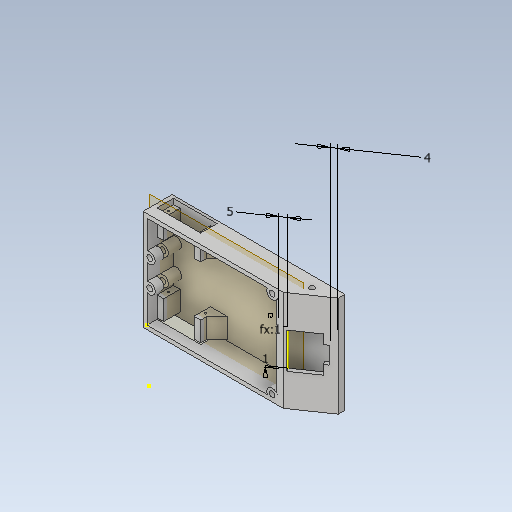
# Autodesk Inventor part: base
Saved by Autodesk Inventor 2020 (Build 240168000, 168)
## iProperties
Created: 2020-01-27
Part Number: base
Material: Ogólne
Document SubType Name: Modeling
Designer: blep
Density: 1 g/cm^3
Appearance: Domyślne
Author: blep
Autodesk Inventor part; units mm, degrees
ref_plane "YZ Plane" through (0, 0, 0) normal (1, 0, 0) x (0, 1, 0)
ref_plane "XZ Plane" through (0, 0, 0) normal (0, 1, 0) x (-1, 0, 0)
sketch "Sketch1" plane through (0, 0, 0) normal (0, 0, 1) x (1, 0, 0)
  line L0 (0, 0) -> (100, 0)
  line L1 (100, 0) -> (100, 70)
  line L2 (100, 70) -> (0, 70)
  line L3 (0, 70) -> (0, 0)
  line L4 (-3, 73) -> (103, 73)
  line L5 (103, 73) -> (103, -3)
  line L6 (103, -3) -> (-3, -3)
  line L7 (-3, -3) -> (-3, 73)
  line L8 (100, 0) -> (103, 0)
  line L9 (100, 70) -> (103, 70)
  dimension "d0" = 100
  dimension "d1" = 70
  dimension "d2" = 3
  constraints: 20 end point, 4 parallel, 3 perpendicular, 2 horizontal, 2 point on line, 3 other
  measures "d0" distance of L2.end L1.end
  measures "d1" distance of L1.end L0.end
  measures "d2" distance between parallel lines of L2 L4
extrude "Extrusion1" add sketch "Sketch1" against normal blind 2
extrude "Extrusion2" add sketch "Sketch1" along normal blind 20 contours L0 L8 L5 L6 L7 L4 L9 L2 L3 | L1 L9 L5 L8
sketch "Sketch2" plane through (0, 70, 0) normal (0, -1, 0) x (1, 0, 0)
  line L0 (0, 0) -> (0, 20) projected
  line L1 (100, 0) -> (0, 0) projected
  line L2 (0, 0) -> (33, 0)
  line L3 (33, 0) -> (33, 12.4)
  line L4 (33, 12.4) -> (0, 12.4)
  line L5 (0, 12.4) -> (0, 0)
  line L6 (100, 0) -> (0, 0) projected
  dimension "d7" = 33
  dimension "d8" = 12.4
  constraints: 8 end point, 2 collinear, 2 parallel, 1 horizontal, 1 perpendicular
  measures "d7" distance of L4.end L3.end
  measures "d8" distance of L3.end L2.end
extrude "Extrusion3" cut sketch "Sketch2" along normal through all both and the other way through all
sketch "Sketch3" plane through (0, 0, 0) normal (0, 0, 1) x (1, 0, 0)
  line L0 (33, 1) -> (28, 1) projected
  line L1 (28, 4) -> (28, 1) projected
  line L2 (0, 1) -> (5, 1) projected
  line L3 (5, 4) -> (5, 1) projected
  line L4 (5, 66) -> (5, 69) projected
  line L5 (0, 69) -> (5, 69) projected
  line L6 (33, 69) -> (28, 69) projected
  line L7 (28, 66) -> (28, 69) projected
  line L8 (33, 54) -> (28, 54)
  line L9 (28, 54) -> (28, 69)
  line L10 (28, 69) -> (33, 69)
  line L11 (33, 69) -> (33, 54)
  line L12 (5, 69) -> (0, 69)
  line L13 (0, 69) -> (0, 54)
  line L14 (0, 54) -> (5, 54)
  line L15 (5, 54) -> (5, 69)
  line L16 (0, 73) -> (0, -3) projected
  line L17 (0, 1) -> (5, 1)
  line L18 (5, 1) -> (5, 16)
  line L19 (5, 16) -> (0, 16)
  line L20 (0, 16) -> (0, 1)
  line L21 (33, 16) -> (28, 16)
  line L22 (28, 16) -> (28, 1)
  line L23 (28, 1) -> (33, 1)
  line L24 (33, 1) -> (33, 16)
  point P0 (0, 0)
  dimension "d11" = 15
  dimension "d12" = 15
  dimension "d13" = 15
  dimension "d14" = 15
  constraints: 32 end point, 8 parallel, 7 collinear, 4 horizontal, 4 perpendicular, 1 coincident, 1 point on line
  measures "d11" distance of L10.end L8.start
  measures "d12" distance of L12.end L13.end
  measures "d13" distance of L17.end L18.end
  measures "d14" distance of L23.end L21.start
ref_plane "Work Plane1" through (0, 66, 12.4) normal (0, 0, 1) x (1, 0, 0)
extrude "Extrusion4" add sketch "Sketch3" along normal up to surface (12.4 mm away)
sketch "Sketch4" plane through (28, 69, 0) normal (0, 1, 0) x (1, 0, 0)
  arc A0 (3.1614, -5.45) -> (3.1614, -6.95) centre (2.5, -6.2) ccw projected
  arc A1 (-26.1614, -6.95) -> (-26.1614, -5.45) centre (-25.5, -6.2) ccw projected
  point P0 (-28, 0)
hole "Hole1" at (30.5, 69, 6.2) at (2.5, 69, 6.2) direction (0, -1, 0) diameter 1.5 end through all
sketch "Sketch5" plane through (-3, 73, -2) normal (0, 1, 0) x (1, 0, 0)
  line L0 (106, -22) -> (0, -22) projected
  line L1 (106, -22) -> (106, 0) projected
  line L2 (0, 0) -> (106, 0) projected
  line L3 (106, -22) -> (106, 0) projected
  line L4 (106, -22) -> (130.7184, -5)
  line L5 (130.7184, -5) -> (130.7184, 0)
  line L6 (130.7184, 0) -> (106, 0)
  line L7 (104.4953, -19.3938) -> (127.7184, -3.4222)
  line L8 (127.7184, -3.4222) -> (127.7184, -3)
  line L9 (127.7184, -3) -> (106, -3)
  line L10 (106, -3) -> (106, 0)
  line L11 (106, -22) -> (100.7059, -22)
  line L12 (100.7059, -22) -> (104.4953, -19.3938)
  point P0 (3, -2)
  dimension "d32" = 30
  dimension "d33" = 5
  dimension "d42" = 3
  constraints: 18 end point, 2 collinear, 2 horizontal, 1 vertical, 2 other
  measures "d32" distance of L0.start L4.end
  measures "d33" distance of L4.end L5.end
  measures "d42" distance between parallel lines of L4 L7
extrude "Extrusion5" cut sketch "Sketch1" along normal through all contours L1 L9 L5 L8
extrude "Extrusion6" add sketch "Sketch5" against normal blind 76 contours L0 L12 L7 L1 | L1 L7 L8 L9 L6 L5 L4
extrude "Extrusion7" add sketch "Sketch5" against normal blind 3 contours L1 L7 L8 L9 L6 L5 L4 | L1 L9 L8 L7
sketch "Sketch6" plane through (-3, -3, -2) normal (0, -1, 0) x (1, 0, 0)
  line L0 (0, 0) -> (130.7184, 0) projected
  line L1 (130.7184, 5) -> (130.7184, 0) projected
  line L2 (106, 22) -> (130.7184, 5) projected
  line L3 (106, 22) -> (106, 0) projected
  point P0 (3, 2)
extrude "Extrusion8" add sketch "Sketch6" against normal blind 3
sketch "Sketch7" plane through (103, 0, 1) normal (-1, 0, 0) x (0, 0, 1)
  line L0 (-1, 0) -> (0, 0) projected
  line L1 (0, 70) -> (0, 0) projected
  line L2 (0, 70) -> (-1, 70) projected
  line L3 (-1, 70) -> (-1, 0) projected
  point P0 (-1, 0)
extrude "Extrusion9" cut sketch "Sketch7" against normal blind 21.75
sketch "Sketch8" plane through (127.7184, -3, 3) normal (0.5667, 0, 0.8239) x (0.8239, 0, -0.5667)
  line L0 (-28, 24.5) -> (-8, 24.5)
  line L1 (-8, 24.5) -> (-8, 51.5)
  line L2 (-8, 51.5) -> (-28, 51.5)
  line L3 (-28, 51.5) -> (-28, 24.5)
  line L4 (0, 76) -> (0, 0) projected
  line L5 (-30, 76) -> (0, 76) projected
  line L6 (-30, 0) -> (-30, 76) projected
  line L7 (0, 0) -> (-30, 0) projected
  line L8 (-28, 51.5) -> (-30, 76) construction
  line L9 (-30, 0) -> (-30, 76) construction
  line L10 (-28, 24.5) -> (-30, 0) construction
  line L11 (-8, 31.5) -> (-5, 31.5)
  line L12 (-5, 31.5) -> (-5, 44.5)
  line L13 (-5, 44.5) -> (-8, 44.5)
  line L14 (-8, 44.5) -> (-8, 31.5)
  line L15 (-8, 24.5) -> (-5, 31.5) construction
  line L16 (-5, 44.5) -> (-8, 51.5) construction
  point P0 (-103.5332, 3)
  dimension "d52" = 27
  dimension "d53" = 20
  dimension "d54" = 3
  dimension "d55" = 13
  dimension "d58" = 2
  constraints: 24 end point, 4 parallel, 2 equal length, 2 horizontal, 2 perpendicular, 1 collinear
  measures "d52" distance of L2.end L0.start
  measures "d53" distance of L1.end L2.end
  measures "d54" distance of L13.end L12.end
  measures "d55" distance of L12.end L11.end
  measures "d58" distance between parallel lines of L9 L3
extrude "Extrusion10" cut sketch "Sketch8" against normal blind 3 contours L3 L2 L1 L0 | L1 L13 L12 L11
sketch "Sketch9" plane through (97.7059, 0, 20) normal (-0.5667, 0, -0.8239) x (-0.8239, 0, 0.5667)
  line L0 (-1.3621, 49.5) -> (-33.3621, 49.5)
  line L1 (-33.3621, 49.5) -> (-33.3621, 20.5)
  line L2 (-33.3621, 20.5) -> (-1.3621, 20.5)
  line L3 (-1.3621, 20.5) -> (-1.3621, 49.5)
  line L4 (-6.3621, 48.5) -> (-6.3621, 21.5) projected
  line L5 (-29.3621, 28.5) -> (-29.3621, 41.5) projected
  point P0 (69.1711, 0)
  dimension "d59" = 5
  dimension "d60" = 4
  dimension "d61" = 1
  dimension "d62" = 1
  constraints: 8 end point, 2 parallel, 1 horizontal, 1 perpendicular
  measures "d59" distance between parallel lines of L3 L4
  measures "d60" distance between parallel lines of L5 L1
  measures "d61" distance from line of L4.end L2
  measures "d62" distance from line of L4.start L0
sketch "Sketch10" plane through (0, 0, 20) normal (0, 0, 1) x (1, 0, 0)
  point P0 (0, 0)
sketch "Sketch12" plane through (-3, -3, -2) normal (0, -1, 0) x (1, 0, 0)
  circle A0 centre (14, 8.2) radius 1.0065 construction
  line L0 (14, 8.2) -> (114, 8.2)
  circle A1 centre (114, 8.2) radius 2
  point P0 (3, 2)
  dimension "d67" = 100
  dimension "d68" = 4
  constraints: 2 end point, 1 centre point, 1 coincident, 1 horizontal
  measures "d67" distance of L0.start L0.end
  measures "d68" diameter of A1
extrude "Extrusion12" cut sketch "Sketch12" against normal through all
sketch "Sketch13" plane through (0, 0, 0) normal (0, 0, 1) x (1, 0, 0)
  circle A0 centre (2, 25) radius 2.125
  circle A1 centre (2, 45) radius 2.125
  line L0 (97.7059, 0) -> (0, 0) projected
  line L1 (0, 70) -> (97.7059, 70) projected
  line L2 (0, 0) -> (0, 70) projected
  circle A2 centre (2, 25) radius 4.125
  circle A3 centre (2, 45) radius 4.125
  dimension "d71" = 25
  dimension "d72" = 25
  dimension "d73" = 2
  dimension "d74" = 4.25
  dimension "d75" = 4.25
  dimension "d76" = 2
  dimension "d77" = 2
  dimension "d78" = 2
  constraints: 4 centre point
  measures "d71" distance from line of L0 A0.centre
  measures "d72" distance from line of L1 A1.centre
  measures "d73" distance from line of A0.centre L2
  measures "d74" diameter of A0
  measures "d75" diameter of A1
  measures "d76" distance from line of A1.centre L2
  measures "d77" radial gap between concentric circles of A0 A2
  measures "d78" radial gap between concentric circles of A1 A3
extrude "Extrusion13" add sketch "Sketch13" along normal up to surface (20 mm away)
extrude "Extrusion14" cut sketch "Sketch13" along normal up to surface (20 mm away) contours A0 L2 | L2 A0 | L2 A1 | A1 L2
sketch "Sketch14" plane through (0, 0, 0) normal (0, 0, 1) x (1, 0, 0)
  circle A0 centre (94.7059, 2) radius 2.125
  circle A1 centre (94.7059, 68) radius 2.125
  circle A2 centre (94.7059, 2) radius 4.125
  circle A3 centre (94.7059, 68) radius 4.125
  line L0 (97.7059, 0) -> (0, 0) projected
  line L1 (33, 70) -> (124.75, 70) projected
  line L2 (97.7059, 70) -> (97.7059, 0) projected
  dimension "d83" = 4.25
  dimension "d84" = 4.25
  dimension "d85" = 2
  dimension "d86" = 2
  dimension "d87" = 2
  dimension "d88" = 2
  dimension "d89" = 3
  dimension "d90" = 3
  constraints: 4 centre point
  measures "d83" diameter of A0
  measures "d84" diameter of A1
  measures "d85" radial gap between concentric circles of A0 A2
  measures "d86" radial gap between concentric circles of A1 A3
  measures "d87" distance from line of L0 A0.centre
  measures "d88" distance from line of L1 A1.centre
  measures "d89" distance from line of L2 A0.centre
  measures "d90" distance from line of L2 A1.centre
extrude "Extrusion15" add sketch "Sketch14" along normal up to surface (20 mm away)
extrude "Extrusion16" cut sketch "Sketch14" along normal up to surface (20 mm away) contours A0 L0 | L0 A0 | L1 A1 | A1 L1
ref_plane "Work Plane2" through (0, 0, 10) normal (0, 0, 1) x (1, 0, 0)
sketch "Sketch15" plane through (0, 0, 10) normal (0, 0, 1) x (1, 0, 0)
  arc A0 (91.0982, 70) -> (98.3136, 70) centre (94.7059, 68) ccw projected
  circle A1 centre (94.7059, 2) radius 4.125
  circle A2 centre (94.7059, 68) radius 4.125
  circle A3 centre (2, 25) radius 4.125
  circle A4 centre (2, 45) radius 4.125
  circle A5 centre (2, 25) radius 2.125 construction
  circle A6 centre (2, 45) radius 2.125 construction
  circle A7 centre (94.7059, 2) radius 2.125 construction
  circle A8 centre (94.7059, 68) radius 2.125 construction
  arc A9 (98.3136, 0) -> (91.0982, 0) centre (94.7059, 2) ccw construction
  arc A10 (0, 21.3923) -> (0, 28.6077) centre (2, 25) ccw construction
  arc A11 (0, 41.3923) -> (0, 48.6077) centre (2, 45) ccw construction
  point P0 (0, 0)
  constraints: 4 centre point, 4 coincident, 4 concentric
extrude "Extrusion17" cut sketch "Sketch15" along normal blind 3.5
chamfer "Chamfer1" distance 8 angle 45 2 edges at (33, 61.5, 0) (33, 8.5, 0)
equation "\"d12\" = d11"
equation "\"d13\" = d11"
equation "\"d14\" = d11"
equation "\"d62\" = d61"
equation "\"d72\" = d71"
equation "\"d75\" = d74"
equation "\"d76\" = d73"
equation "\"d88\" = d87"
equation "\"d90\" = d89"
body "Solid1"
